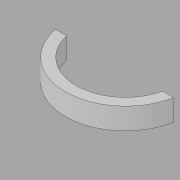
# Autodesk Inventor part: g_jaws
Saved by Autodesk Inventor 2019 (Build 230136000, 136)
## iProperties
Created: 2021-11-03
Part Number: g_jaws
Material: Generic
Document SubType Name: Modeling
Designer: Mohamed
Density: 1 g/cm^3
Appearance: Default
Author: Mohamed
Autodesk Inventor part; units mm, degrees
ref_plane "YZ Plane" through (0, 0, 0) normal (1, 0, 0) x (0, 1, 0)
ref_plane "XZ Plane" through (0, 0, 0) normal (0, 1, 0) x (-1, 0, 0)
ref_plane "XY Plane" through (0, 0, 0) normal (0, 0, 1) x (1, 0, 0)
sketch "Sketch1" plane through (0, 0, 0) normal (0, 1, 0) x (-1, 0, 0)
  line L0 (22.4333, 5.0741) -> (27.5333, 5.0909)
  line L1 (-22.4333, 5.0741) -> (-27.5333, 5.0909)
  arc A0 (22.4333, 5.0741) -> (-22.4333, 5.0741) centre (0, 0) ccw
  arc A1 (27.5333, 5.0909) -> (-27.5333, 5.0909) centre (0, 0) ccw
  constraints: 4 end point, 4 point on circle, 2 centre point, 1 coincident
extrude "Extrusion1" add sketch "Sketch1" along normal blind 10
body "Solid1"
